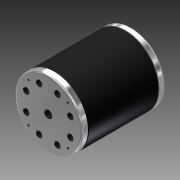
# Autodesk Inventor part: my1020_motor
Saved by Autodesk Inventor 2012 (Build 160160000, 160)
## iProperties
Created: 2012-01-29
Part Number: my1020_motor
Material: Default
Document SubType Name: Modeling
Designer: Antonella Wilby
Density: 1 g/cm^3
Author: Antonella Wilby
Autodesk Inventor part; units mm, degrees
ref_plane "YZ Plane" through (0, 0, 0) normal (1, 0, 0) x (0, 1, 0)
ref_plane "XZ Plane" through (0, 0, 0) normal (0, 1, 0) x (-1, 0, 0)
ref_plane "XY Plane" through (0, 0, 0) normal (0, 0, 1) x (1, 0, 0)
sketch "Sketch1" plane through (0, 0, 0) normal (0, 0, 1) x (1, 0, 0)
  circle A0 centre (0, 0) radius 53.975
  dimension "d0" = 107.95
  constraints: 1 centre point, 1 coincident
  measures "d0" diameter of A0
extrude "Extrusion1" add sketch "Sketch1" along normal mid plane 114.3
chamfer "Chamfer1" distance 1.5875 angle 45 1 edges at (-53.975, 0, 57.15)
chamfer "Chamfer2" distance 1.5875 angle 45 1 edges at (-53.975, 0, -57.15)
sketch "Sketch3" plane through (0, 0, 57.15) normal (0, 0, 1) x (1, 0, 0)
  circle A0 centre (0, 0) radius 53.975 projected
extrude "Front End" add sketch "Sketch3" along normal blind 9.525
sketch "Sketch5" plane through (0, 0, 66.675) normal (0, 0, 1) x (1, 0, 0)
  circle A0 centre (0, 0) radius 53.975 projected
  line L0 (0, 0) -> (31.4309, 31.4309) construction
  line L1 (-75.565, 0) -> (75.565, 0) projected
  line L2 (0, -75.565) -> (0, 75.565) projected
  point P0 (-31.4309, 31.4309)
  point P1 (-31.4309, -31.4309)
  point P2 (31.4309, -31.4309)
  dimension "d25" = 360
  dimension "d46" = 45
  dimension "d47" = 44.45
  constraints: 2 end point, 5 other
  measures "d46" angle of L0 L1
  measures "d47" distance of L0.start L0.end
hole "Mount Holes" at (31.4309, 31.4309, 66.675) at (-31.4309, 31.4309, 66.675) at (-31.4309, -31.4309, 66.675) at (31.4309, -31.4309, 66.675) direction (0, 0, -1) diameter 3.683 depth 12.7 tip angle 118 thread size "10-24 UNC" class "2B" standard "ANSI Unified Screw Threads"
sketch "Sketch6" plane through (0, 0, 66.675) normal (0, 0, 1) x (1, 0, 0)
  circle A0 centre (0, 0) radius 53.975 projected
  circle A1 centre (0, 0) radius 6.35
  dimension "d34" = 12.7
  constraints: 1 centre point, 1 coincident
  measures "d34" diameter of A1
extrude "Shaft Hole" cut sketch "Sketch6" against normal blind 12.7 contours A1
sketch "Sketch7" plane through (0, 0, 66.675) normal (0, 0, 1) x (1, 0, 0)
  circle A0 centre (0, 0) radius 6.35 projected
  circle A1 centre (0, 0) radius 53.975 projected
  circle A2 centre (35.1998, 14.5802) radius 5.08
  line L0 (0, 0) -> (35.1998, 14.5802) construction
  line L1 (0, -75.565) -> (0, 75.565) projected
  line L2 (-75.565, 0) -> (75.565, 0) projected
  circle A3 centre (14.5802, 35.1998) radius 5.08
  circle A4 centre (-14.5802, 35.1998) radius 5.08
  circle A5 centre (-35.1998, 14.5802) radius 5.08
  circle A6 centre (-35.1998, -14.5802) radius 5.08
  circle A7 centre (-14.5802, -35.1998) radius 5.08
  circle A8 centre (14.5802, -35.1998) radius 5.08
  circle A9 centre (35.1998, -14.5802) radius 5.08
  dimension "d37" = 10.16
  dimension "d38" = 22.5
  dimension "d39" = 38.1
  dimension "d42" = 360
  constraints: 8 centre point, 2 end point, 17 other
  measures "d37" diameter of A2
  measures "d38" angle of L0 L2
  measures "d39" distance of L0.start L0.end
extrude "Ventilation Holes" cut sketch "Sketch7" against normal blind 12.7 contours A2 | A3 | A4 | A5 | A6 | A7 | A8 | A9
mirror "Mirror3" about plane through (0, 0, 0) normal (0, 0, 1) of "Front End", "Mount Holes", "Ventilation Holes"
fillet "Fillet1" radius 3.175 2 edges at (-53.975, 0, 66.675) (-53.975, 0, -66.675)
body "Solid1"
